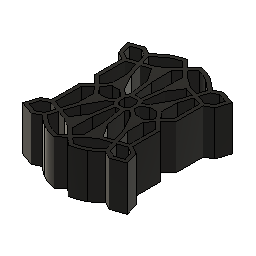
SC-002_shell (Autodesk Fusion 360 design; units mm, degrees)
Autodesk Fusion 360 part; units mm, degrees
sketch "Sketch1" plane through (0, 0, 0) normal (0, 1, 0) x (1, 0, 0)
  line L0 (-3.2742, 2.0082) -> (-1.6589, 0.7858)
  line L1 (-1.6589, 0.7858) -> (-1.6153, -0.6985)
  line L2 (-1.6153, -0.6985) -> (-3.1869, -1.8336)
  line L3 (-3.1869, -1.8336) -> (-5.1951, -1.8336)
  line L4 (-5.1951, -1.8336) -> (-6.8977, 0)
  line L5 (-6.8977, 0) -> (-5.1951, 2.0082)
  line L6 (-5.1951, 2.0082) -> (-3.2742, 2.0082)
  line L7 (3.2742, 2.0082) -> (1.6589, 0.7858)
  line L8 (1.6589, 0.7858) -> (1.6153, -0.6985)
  line L9 (1.6153, -0.6985) -> (3.1869, -1.8336)
  line L10 (3.1869, -1.8336) -> (5.1951, -1.8336)
  line L11 (5.1951, -1.8336) -> (6.8977, 0)
  line L12 (6.8977, 0) -> (5.1951, 2.0082)
  line L13 (5.1951, 2.0082) -> (3.2742, 2.0082)
  line L14 (0, 13.0532) -> (-1.7026, 14.7558)
  spline S0 degree 3 poles (-1.7026, 14.7558) (-2.3211, 14.6321) (-3.7632, 14.197) (-4.6712, 13.5334) knots 0 0 0 0 1 1 1 1
  spline S1 degree 3 poles (-4.6712, 13.5334) (-5.5793, 12.8698) (-6.6576, 11.9181) (-7.0723, 11.5252) knots 0 0 0 0 1 1 1 1
  line L15 (-7.0723, 11.5252) -> (-6.3302, 8.9932)
  line L16 (-6.3302, 8.9932) -> (-3.7544, 9.8663)
  line L17 (-3.7544, 9.8663) -> (-1.7026, 11.3506)
  line L18 (-1.7026, 11.3506) -> (0, 13.0532)
  line L19 (0, 13.0532) -> (1.7026, 14.7558)
  spline S2 degree 3 poles (1.7026, 14.7558) (2.3211, 14.6321) (3.7632, 14.197) (4.6712, 13.5334) knots 0 0 0 0 1 1 1 1
  spline S3 degree 3 poles (4.6712, 13.5334) (5.5793, 12.8698) (6.6576, 11.9181) (7.0723, 11.5252) knots 0 0 0 0 1 1 1 1
  line L20 (7.0723, 11.5252) -> (6.3302, 8.9932)
  line L21 (6.3302, 8.9932) -> (3.7544, 9.8663)
  line L22 (3.7544, 9.8663) -> (1.7026, 11.3506)
  line L23 (1.7026, 11.3506) -> (0, 13.0532)
  line L24 (0, -12.8786) -> (-1.7026, -14.4939)
  spline S4 degree 3 poles (-1.7026, -14.4939) (-2.3211, -14.3702) (-3.689, -14.0355) (-4.6712, -13.4462) knots 0 0 0 0 1 1 1 1
  spline S5 degree 3 poles (-4.6712, -13.4462) (-5.6356, -12.8675) (-6.6576, -11.9182) (-7.0723, -11.5253) knots 0 0 0 0 1 1 1 1
  line L25 (-7.0723, -11.5253) -> (-6.3302, -8.9932)
  line L26 (-6.3302, -8.9932) -> (-3.7544, -9.8663)
  line L27 (-3.7544, -9.8663) -> (-1.7026, -11.176)
  line L28 (-1.7026, -11.176) -> (0, -12.8786)
  line L29 (0, -12.8786) -> (1.7026, -14.4939)
  spline S6 degree 3 poles (1.7026, -14.4939) (2.3211, -14.3702) (3.689, -14.0355) (4.6712, -13.4462) knots 0 0 0 0 1 1 1 1
  spline S7 degree 3 poles (4.6712, -13.4462) (5.6356, -12.8675) (6.6576, -11.9182) (7.0723, -11.5253) knots 0 0 0 0 1 1 1 1
  line L30 (7.0723, -11.5253) -> (6.3302, -8.9932)
  line L31 (6.3302, -8.9932) -> (3.7544, -9.8663)
  line L32 (3.7544, -9.8663) -> (1.7026, -11.176)
  line L33 (1.7026, -11.176) -> (0, -12.8786)
  line L34 (0, 13.0532) -> (-1.7026, 11.3506)
  line L35 (-1.7026, 11.3506) -> (-1.6153, 6.5921)
  line L36 (-1.6153, 6.5921) -> (-1.0041, 1.9645)
  line L37 (-1.0041, 1.9645) -> (0, 1.9645)
  line L38 (0, 1.9645) -> (1.0041, 1.9645)
  line L39 (1.0041, 1.9645) -> (1.6153, 6.5921)
  line L40 (1.6153, 6.5921) -> (1.7026, 11.3506)
  line L41 (1.7026, 11.3506) -> (0, 13.0532)
  line L42 (0, -12.8786) -> (-1.7026, -11.176)
  line L43 (-1.7026, -11.176) -> (-1.6153, -6.5921)
  line L44 (-1.6153, -6.5921) -> (-0.8731, -1.7899)
  line L45 (-0.8731, -1.7899) -> (0, -1.7899)
  line L46 (0, -1.7899) -> (0.8731, -1.7899)
  line L47 (0.8731, -1.7899) -> (1.6153, -6.5921)
  line L48 (1.6153, -6.5921) -> (1.7026, -11.176)
  line L49 (1.7026, -11.176) -> (0, -12.8786)
  line L50 (0, 1.9645) -> (-1.0041, 1.9645)
  line L51 (-1.0041, 1.9645) -> (-1.6589, 0.7858)
  line L52 (-1.6589, 0.7858) -> (-1.6153, -0.6985)
  line L53 (-1.6153, -0.6985) -> (-0.8731, -1.7899)
  line L54 (-0.8731, -1.7899) -> (0, -1.7899)
  line L55 (0, -1.7899) -> (0.8731, -1.7899)
  line L56 (0.8731, -1.7899) -> (1.6153, -0.6985)
  line L57 (1.6153, -0.6985) -> (1.6589, 0.7858)
  line L58 (1.6589, 0.7858) -> (1.0041, 1.9645)
  line L59 (1.0041, 1.9645) -> (0, 1.9645)
  line L60 (-1.6589, 0.7858) -> (-1.0041, 1.9645)
  line L61 (-1.0041, 1.9645) -> (-1.6153, 6.5921)
  line L62 (-1.6153, 6.5921) -> (-3.7544, 9.8663)
  line L63 (-3.7544, 9.8663) -> (-6.3302, 8.9932)
  line L64 (-6.3302, 8.9932) -> (-5.2388, 5.6316)
  line L65 (-5.2388, 5.6316) -> (-3.2742, 2.0082)
  line L66 (-3.2742, 2.0082) -> (-1.6589, 0.7858)
  line L67 (1.6589, 0.7858) -> (1.0041, 1.9645)
  line L68 (1.0041, 1.9645) -> (1.6153, 6.5921)
  line L69 (1.6153, 6.5921) -> (3.7544, 9.8663)
  line L70 (3.7544, 9.8663) -> (6.3302, 8.9932)
  line L71 (6.3302, 8.9932) -> (5.2387, 5.6316)
  line L72 (5.2387, 5.6316) -> (3.2742, 2.0082)
  line L73 (3.2742, 2.0082) -> (1.6589, 0.7858)
  line L74 (-1.6153, -0.6985) -> (-0.8731, -1.7899)
  line L75 (-0.8731, -1.7899) -> (-1.6153, -6.5921)
  line L76 (-1.6153, -6.5921) -> (-3.7544, -9.8663)
  line L77 (-3.7544, -9.8663) -> (-6.3302, -8.9932)
  line L78 (-6.3302, -8.9932) -> (-5.2388, -5.6317)
  line L79 (-5.2388, -5.6317) -> (-3.1869, -1.8336)
  line L80 (-3.1869, -1.8336) -> (-1.6153, -0.6985)
  line L81 (1.6153, -0.6985) -> (0.8731, -1.7899)
  line L82 (0.8731, -1.7899) -> (1.6153, -6.5921)
  line L83 (1.6153, -6.5921) -> (3.7544, -9.8663)
  line L84 (3.7544, -9.8663) -> (6.3302, -8.9932)
  line L85 (6.3302, -8.9932) -> (5.2387, -5.6317)
  line L86 (5.2387, -5.6317) -> (3.1869, -1.8336)
  line L87 (3.1869, -1.8336) -> (1.6153, -0.6985)
  line L88 (-8.8186, 12.442) -> (-7.0723, 11.5252)
  line L89 (-7.0723, 11.5252) -> (-6.3302, 8.9932)
  line L90 (-6.3302, 8.9932) -> (-8.7749, 8.1637)
  line L91 (-8.7749, 8.1637) -> (-10.5212, 9.1241)
  line L92 (-10.5212, 9.1241) -> (-11.307, 11.5689)
  line L93 (-11.307, 11.5689) -> (-8.8186, 12.442)
  line L94 (8.8186, 12.442) -> (7.0723, 11.5252)
  line L95 (7.0723, 11.5252) -> (6.3302, 8.9932)
  line L96 (6.3302, 8.9932) -> (8.7749, 8.1637)
  line L97 (8.7749, 8.1637) -> (10.5212, 9.1241)
  line L98 (10.5212, 9.1241) -> (11.307, 11.5689)
  line L99 (11.307, 11.5689) -> (8.8186, 12.442)
  line L100 (-8.8186, -12.4421) -> (-7.0723, -11.5253)
  line L101 (-7.0723, -11.5253) -> (-6.3302, -8.9932)
  line L102 (-6.3302, -8.9932) -> (-8.7749, -8.1637)
  line L103 (-8.7749, -8.1637) -> (-10.5212, -9.1242)
  line L104 (-10.5212, -9.1242) -> (-11.307, -11.5689)
  line L105 (-11.307, -11.5689) -> (-8.8186, -12.4421)
  line L106 (8.8186, -12.4421) -> (7.0723, -11.5253)
  line L107 (7.0723, -11.5253) -> (6.3302, -8.9932)
  line L108 (6.3302, -8.9932) -> (8.7749, -8.1637)
  line L109 (8.7749, -8.1637) -> (10.5212, -9.1242)
  line L110 (10.5212, -9.1242) -> (11.307, -11.5689)
  line L111 (11.307, -11.5689) -> (8.8186, -12.4421)
  line L112 (-8.7749, 8.1637) -> (-6.3302, 8.9932)
  line L113 (-6.3302, 8.9932) -> (-5.2388, 5.6316)
  line L114 (-5.2388, 5.6316) -> (-5.1951, 2.0082)
  line L115 (-5.1951, 2.0082) -> (-6.8977, 0)
  line L116 (-6.8977, 0) -> (-8.7749, 1.9208)
  line L117 (-8.7749, 1.9208) -> (-8.7749, 8.1637)
  line L118 (8.7749, 8.1637) -> (6.3302, 8.9932)
  line L119 (6.3302, 8.9932) -> (5.2387, 5.6316)
  line L120 (5.2387, 5.6316) -> (5.1951, 2.0082)
  line L121 (5.1951, 2.0082) -> (6.8977, 0)
  line L122 (6.8977, 0) -> (8.7749, 1.9208)
  line L123 (8.7749, 1.9208) -> (8.7749, 8.1637)
  line L124 (-8.7749, -8.1637) -> (-6.3302, -8.9932)
  line L125 (-6.3302, -8.9932) -> (-5.2388, -5.6317)
  line L126 (-5.2388, -5.6317) -> (-5.1951, -1.8336)
  line L127 (-5.1951, -1.8336) -> (-6.8977, 0)
  line L128 (-6.8977, 0) -> (-8.7749, -1.9209)
  line L129 (-8.7749, -1.9209) -> (-8.7749, -8.1637)
  line L130 (8.7749, -8.1637) -> (6.3302, -8.9932)
  line L131 (6.3302, -8.9932) -> (5.2387, -5.6317)
  line L132 (5.2387, -5.6317) -> (5.1951, -1.8336)
  line L133 (5.1951, -1.8336) -> (6.8977, 0)
  line L134 (6.8977, 0) -> (8.7749, -1.9209)
  line L135 (8.7749, -1.9209) -> (8.7749, -8.1637)
  line L136 (0, 0) -> (0, 13.0532)
  constraint coincident L136.start origin
sketch "Sketch2" plane through (0, 0, 0) normal (0, 1, 0) x (1, 0, 0)
  line L0 (0, 0) -> (0, 15)
  line L1 (7.5, 15) -> (-7.5, 15)
  line L2 (-7.5, 15) -> (-7.5, -15)
  line L3 (-7.5, -15) -> (7.5, -15)
  line L4 (7.5, -15) -> (7.5, 15)
  line L5 (7.5, 15) -> (-7.5, -15) construction
  line L6 (-7.5, 15) -> (7.5, -15) construction
  dimension "d2" = 15
  dimension "d4" = 15
  dimension "d5" = 30
  constraint coincident L0.start origin
  constraint vertical L0
  constraint horizontal L1
  constraint perpendicular L1 L2
  constraint parallel L1 L3
  constraint parallel L2 L4
  constraint coincident L5 L0.start
  constraint coincident L6 L0.start
  measures "d2" distance of L0.start L0.end
  measures "d4" distance of L2.end L3.end
  measures "d5" distance of L1.end L2.end
scale "Scale1" [no effect]
sketch "Sketch3" plane through (0, 0, 0) normal (0, 1, 0) x (1, 0, 0)
  line L0 (-11.307, 11.5689) -> (-8.8186, 12.442)
  line L1 (-8.8186, 12.442) -> (-7.0723, 11.5252)
  spline S0 degree 3 poles (-4.6712, 13.5334) (-5.5793, 12.8698) (-6.6576, 11.9181) (-7.0723, 11.5252) knots 0 0 0 0 1 1 1 1
  spline S1 degree 3 poles (-1.7026, 14.7558) (-2.3211, 14.6321) (-3.7632, 14.197) (-4.6712, 13.5334) knots 0 0 0 0 1 1 1 1
  line L2 (0, 13.0532) -> (-1.7026, 14.7558)
  line L3 (0, 13.0532) -> (1.7026, 14.7558)
  spline S2 degree 3 poles (1.7026, 14.7558) (2.3211, 14.6321) (3.7632, 14.197) (4.6712, 13.5334) knots 0 0 0 0 1 1 1 1
  spline S3 degree 3 poles (4.6712, 13.5334) (5.5793, 12.8698) (6.6576, 11.9181) (7.0723, 11.5252) knots 0 0 0 0 1 1 1 1
  line L4 (8.8186, 12.442) -> (7.0723, 11.5252)
  line L5 (11.307, 11.5689) -> (8.8186, 12.442)
  line L6 (10.5212, 9.1241) -> (11.307, 11.5689)
  line L7 (8.7749, 8.1637) -> (10.5212, 9.1241)
  line L8 (8.7749, 1.9208) -> (8.7749, 8.1637)
  line L9 (6.8977, 0) -> (8.7749, 1.9208)
  line L10 (6.8977, 0) -> (8.7749, -1.9209)
  line L11 (8.7749, -1.9209) -> (8.7749, -8.1637)
  line L12 (8.7749, -8.1637) -> (10.5212, -9.1242)
  line L13 (10.5212, -9.1242) -> (11.307, -11.5689)
  line L14 (11.307, -11.5689) -> (8.8186, -12.4421)
  line L15 (8.8186, -12.4421) -> (7.0723, -11.5253)
  spline S4 degree 3 poles (4.6712, -13.4462) (5.6356, -12.8675) (6.6576, -11.9182) (7.0723, -11.5253) knots 0 0 0 0 1 1 1 1
  spline S5 degree 3 poles (1.7026, -14.4939) (2.3211, -14.3702) (3.689, -14.0355) (4.6712, -13.4462) knots 0 0 0 0 1 1 1 1
  line L16 (0, -12.8786) -> (1.7026, -14.4939)
  line L17 (0, -12.8786) -> (-1.7026, -14.4939)
  spline S6 degree 3 poles (-1.7026, -14.4939) (-2.3211, -14.3702) (-3.689, -14.0355) (-4.6712, -13.4462) knots 0 0 0 0 1 1 1 1
  spline S7 degree 3 poles (-4.6712, -13.4462) (-5.6356, -12.8675) (-6.6576, -11.9182) (-7.0723, -11.5253) knots 0 0 0 0 1 1 1 1
  line L18 (-8.8186, -12.4421) -> (-7.0723, -11.5253)
  line L19 (-11.307, -11.5689) -> (-8.8186, -12.4421)
  line L20 (-10.5212, -9.1242) -> (-11.307, -11.5689)
  line L21 (-8.7749, -8.1637) -> (-10.5212, -9.1242)
  line L22 (-8.7749, -1.9209) -> (-8.7749, -8.1637)
  line L23 (-6.8977, 0) -> (-8.7749, -1.9209)
  line L24 (-6.8977, 0) -> (-8.7749, 1.9208)
  line L25 (-8.7749, 1.9208) -> (-8.7749, 8.1637)
  line L26 (-8.7749, 8.1637) -> (-10.5212, 9.1241)
  line L27 (-10.5212, 9.1241) -> (-11.307, 11.5689)
  line L28 (-8.7749, 8.1637) -> (-6.3302, 8.9932)
  line L29 (-7.0723, 11.5252) -> (-6.3302, 8.9932)
  line L30 (-6.3302, 8.9932) -> (-3.7544, 9.8663)
  line L31 (-3.7544, 9.8663) -> (-1.7026, 11.3506)
  line L32 (0, 13.0532) -> (-1.7026, 11.3506)
  line L33 (1.7026, 11.3506) -> (0, 13.0532)
  line L34 (3.7544, 9.8663) -> (1.7026, 11.3506)
  line L35 (3.7544, 9.8663) -> (6.3302, 8.9932)
  line L36 (7.0723, 11.5252) -> (6.3302, 8.9932)
  line L37 (6.3302, 8.9932) -> (8.7749, 8.1637)
  line L38 (6.3302, -8.9932) -> (8.7749, -8.1637)
  line L39 (7.0723, -11.5253) -> (6.3302, -8.9932)
  line L40 (3.7544, -9.8663) -> (6.3302, -8.9932)
  line L41 (3.7544, -9.8663) -> (1.7026, -11.176)
  line L42 (1.7026, -11.176) -> (0, -12.8786)
  line L43 (0, -12.8786) -> (-1.7026, -11.176)
  line L44 (-3.7544, -9.8663) -> (-1.7026, -11.176)
  line L45 (-3.7544, -9.8663) -> (-6.3302, -8.9932)
  line L46 (-7.0723, -11.5253) -> (-6.3302, -8.9932)
  line L47 (-6.3302, -8.9932) -> (-8.7749, -8.1637)
  line L48 (-6.3302, -8.9932) -> (-5.2388, -5.6317)
  line L49 (-5.2388, -5.6317) -> (-3.1869, -1.8336)
  line L50 (-5.2388, -5.6317) -> (-5.1951, -1.8336)
  line L51 (-5.1951, -1.8336) -> (-6.8977, 0)
  line L52 (-3.1869, -1.8336) -> (-5.1951, -1.8336)
  line L53 (-5.1951, 2.0082) -> (-6.8977, 0)
  line L54 (-5.2388, 5.6316) -> (-5.1951, 2.0082)
  line L55 (-6.3302, 8.9932) -> (-5.2388, 5.6316)
  line L56 (-5.1951, 2.0082) -> (-3.2742, 2.0082)
  line L57 (-5.2388, 5.6316) -> (-3.2742, 2.0082)
  line L58 (-3.2742, 2.0082) -> (-1.6589, 0.7858)
  line L59 (-1.0041, 1.9645) -> (-1.6153, 6.5921)
  line L60 (-1.6153, 6.5921) -> (-3.7544, 9.8663)
  line L61 (-1.7026, 11.3506) -> (-1.6153, 6.5921)
  line L62 (1.6153, 6.5921) -> (1.7026, 11.3506)
  line L63 (1.6153, 6.5921) -> (3.7544, 9.8663)
  line L64 (6.3302, 8.9932) -> (5.2387, 5.6316)
  line L65 (5.2387, 5.6316) -> (5.1951, 2.0082)
  line L66 (5.1951, 2.0082) -> (6.8977, 0)
  line L67 (5.1951, -1.8336) -> (6.8977, 0)
  line L68 (5.2387, -5.6317) -> (5.1951, -1.8336)
  line L69 (6.3302, -8.9932) -> (5.2387, -5.6317)
  line L70 (1.6153, -6.5921) -> (3.7544, -9.8663)
  line L71 (1.6153, -6.5921) -> (1.7026, -11.176)
  line L72 (-1.7026, -11.176) -> (-1.6153, -6.5921)
  line L73 (-1.6153, -6.5921) -> (-3.7544, -9.8663)
  line L74 (-1.6153, -6.5921) -> (-0.8731, -1.7899)
  line L75 (0.8731, -1.7899) -> (1.6153, -6.5921)
  line L76 (5.2387, -5.6317) -> (3.1869, -1.8336)
  line L77 (3.1869, -1.8336) -> (5.1951, -1.8336)
  line L78 (0, -1.7899) -> (0.8731, -1.7899)
  line L79 (-1.6153, -0.6985) -> (-3.1869, -1.8336)
  line L80 (-1.6153, -0.6985) -> (-0.8731, -1.7899)
  line L81 (-0.8731, -1.7899) -> (0, -1.7899)
  line L82 (0.8731, -1.7899) -> (1.6153, -0.6985)
  line L83 (1.6153, -0.6985) -> (3.1869, -1.8336)
  line L84 (1.6589, 0.7858) -> (1.6153, -0.6985)
  line L85 (-1.6589, 0.7858) -> (-1.6153, -0.6985)
  line L86 (-1.6589, 0.7858) -> (-1.0041, 1.9645)
  line L87 (0, 1.9645) -> (-1.0041, 1.9645)
  line L88 (1.0041, 1.9645) -> (0, 1.9645)
  line L89 (1.6589, 0.7858) -> (1.0041, 1.9645)
  line L90 (1.0041, 1.9645) -> (1.6153, 6.5921)
  line L91 (3.2742, 2.0082) -> (1.6589, 0.7858)
  line L92 (5.1951, 2.0082) -> (3.2742, 2.0082)
  line L93 (5.2387, 5.6316) -> (3.2742, 2.0082)
  line L94 (-7.4085, 11.2499) -> (-6.8219, 9.2487)
  line L95 (-8.7365, 8.5991) -> (-6.8219, 9.2487)
  line L96 (-8.7365, 8.5991) -> (-10.189, 9.398)
  line L97 (-10.189, 9.398) -> (-10.807, 11.3204)
  line L98 (-10.807, 11.3204) -> (-8.8504, 12.0069)
  line L99 (-8.8504, 12.0069) -> (-7.4085, 11.2499)
  line L100 (-0.5657, 13.0532) -> (-1.9629, 11.656)
  line L101 (-3.94, 10.2257) -> (-1.9629, 11.656)
  line L102 (-6.0636, 9.5059) -> (-3.94, 10.2257)
  line L103 (-6.6189, 11.4005) -> (-6.0636, 9.5059)
  spline S8 degree 3 poles (-4.4352, 13.2105) (-5.2085, 12.6454) (-6.1342, 11.8442) (-6.6189, 11.4005) knots 0 0 0 0 0.875986 0.875986 0.875986 0.875986
  spline S9 degree 3 poles (-1.8301, 14.3176) (-2.4821, 14.1594) (-3.7085, 13.7415) (-4.4352, 13.2105) knots 0.105546 0.105546 0.105546 0.105546 1 1 1 1
  line L104 (-0.5657, 13.0532) -> (-1.8301, 14.3176)
  line L105 (1.9629, 11.656) -> (0.5657, 13.0532)
  line L106 (0.5657, 13.0532) -> (1.8301, 14.3176)
  spline S10 degree 3 poles (1.8301, 14.3176) (2.4821, 14.1594) (3.7085, 13.7415) (4.4352, 13.2105) knots 0.105546 0.105546 0.105546 0.105546 1 1 1 1
  spline S11 degree 3 poles (4.4352, 13.2105) (5.2085, 12.6454) (6.1342, 11.8442) (6.6189, 11.4005) knots 0 0 0 0 0.875986 0.875986 0.875986 0.875986
  line L107 (6.6189, 11.4005) -> (6.0636, 9.5059)
  line L108 (3.94, 10.2257) -> (6.0636, 9.5059)
  line L109 (3.94, 10.2257) -> (1.9629, 11.656)
  line L110 (6.8219, 9.2487) -> (8.7365, 8.5991)
  line L111 (8.7365, 8.5991) -> (10.189, 9.398)
  line L112 (10.189, 9.398) -> (10.8069, 11.3204)
  line L113 (10.8069, 11.3204) -> (8.8504, 12.0069)
  line L114 (8.8504, 12.0069) -> (7.4084, 11.2499)
  line L115 (7.4084, 11.2499) -> (6.8219, 9.2487)
  line L116 (6.5854, 8.4841) -> (8.3749, 7.877)
  line L117 (8.3749, 2.0838) -> (8.3749, 7.877)
  line L118 (6.9187, 0.5938) -> (8.3749, 2.0838)
  line L119 (5.5969, 2.1528) -> (6.9187, 0.5938)
  line L120 (5.638, 5.566) -> (5.5969, 2.1528)
  line L121 (6.5854, 8.4841) -> (5.638, 5.566)
  line L122 (1.418, 2.0432) -> (1.9999, 6.4495)
  line L123 (1.9999, 6.4495) -> (3.9197, 9.3879)
  line L124 (3.9197, 9.3879) -> (5.8278, 8.7411)
  line L125 (5.8278, 8.7411) -> (4.8696, 5.79)
  line L126 (4.8696, 5.79) -> (2.9638, 2.2749)
  line L127 (2.9638, 2.2749) -> (1.7849, 1.3827)
  line L128 (1.7849, 1.3827) -> (1.418, 2.0432)
  line L129 (1.2995, 11.188) -> (0, 12.4875)
  line L130 (0, 12.4875) -> (-1.2995, 11.188)
  line L131 (-1.2995, 11.188) -> (-1.2158, 6.622)
  line L132 (-0.6535, 2.3645) -> (-1.2158, 6.622)
  line L133 (0, 2.3645) -> (-0.6535, 2.3645)
  line L134 (0.6534, 2.3645) -> (0, 2.3645)
  line L135 (0.6534, 2.3645) -> (1.2158, 6.622)
  line L136 (1.2158, 6.622) -> (1.2995, 11.188)
  line L137 (-1.2559, 0.6876) -> (-0.7687, 1.5645)
  line L138 (0, 1.5645) -> (-0.7687, 1.5645)
  line L139 (0.7687, 1.5645) -> (0, 1.5645)
  line L140 (1.2559, 0.6876) -> (0.7687, 1.5645)
  line L141 (1.2559, 0.6876) -> (1.2189, -0.5701)
  line L142 (0.6614, -1.3899) -> (1.2189, -0.5701)
  line L143 (0, -1.3899) -> (0.6614, -1.3899)
  line L144 (-0.6614, -1.3899) -> (0, -1.3899)
  line L145 (-1.2189, -0.5701) -> (-0.6614, -1.3899)
  line L146 (-1.2559, 0.6876) -> (-1.2189, -0.5701)
  line L147 (-1.9999, 6.4495) -> (-3.9197, 9.3879)
  line L148 (-5.8278, 8.7411) -> (-3.9197, 9.3879)
  line L149 (-5.8278, 8.7411) -> (-4.8696, 5.79)
  line L150 (-4.8696, 5.79) -> (-2.9638, 2.2749)
  line L151 (-2.9638, 2.2749) -> (-1.7849, 1.3827)
  line L152 (-1.7849, 1.3827) -> (-1.418, 2.0432)
  line L153 (-1.418, 2.0432) -> (-1.9999, 6.4495)
  line L154 (-6.5854, 8.4841) -> (-5.638, 5.566)
  line L155 (-5.638, 5.566) -> (-5.5969, 2.1528)
  line L156 (-5.5969, 2.1528) -> (-6.9187, 0.5938)
  line L157 (-6.9187, 0.5938) -> (-8.3749, 2.0838)
  line L158 (-8.3749, 2.0838) -> (-8.3749, 7.877)
  line L159 (-8.3749, 7.877) -> (-6.5854, 8.4841)
  line L160 (-2.0531, 0.5825) -> (-2.0213, -0.4984)
  line L161 (-2.0213, -0.4984) -> (-3.3163, -1.4336)
  line L162 (-3.3163, -1.4336) -> (-5.0207, -1.4336)
  line L163 (-5.0207, -1.4336) -> (-6.363, 0.012)
  line L164 (-5.0098, 1.6082) -> (-6.363, 0.012)
  line L165 (-5.0098, 1.6082) -> (-3.4085, 1.6082)
  line L166 (-3.4085, 1.6082) -> (-2.0531, 0.5825)
  line L167 (5.0098, 1.6082) -> (3.4085, 1.6082)
  line L168 (3.4085, 1.6082) -> (2.0531, 0.5825)
  line L169 (2.0531, 0.5825) -> (2.0213, -0.4984)
  line L170 (2.0213, -0.4984) -> (3.3162, -1.4336)
  line L171 (3.3162, -1.4336) -> (5.0207, -1.4336)
  line L172 (5.0207, -1.4336) -> (6.363, 0.012)
  line L173 (5.0098, 1.6082) -> (6.363, 0.012)
  line L174 (6.9051, -0.5799) -> (8.3749, -2.0839)
  line L175 (8.3749, -2.0839) -> (8.3749, -7.8771)
  line L176 (6.5854, -8.4842) -> (8.3749, -7.8771)
  line L177 (6.5854, -8.4842) -> (5.638, -5.5661)
  line L178 (5.638, -5.5661) -> (5.5969, -1.9887)
  line L179 (5.5969, -1.9887) -> (6.9051, -0.5799)
  line L180 (8.7365, -8.5992) -> (10.189, -9.398)
  line L181 (10.189, -9.398) -> (10.8069, -11.3205)
  line L182 (10.8069, -11.3205) -> (8.8504, -12.007)
  line L183 (8.8504, -12.007) -> (7.4084, -11.25)
  line L184 (7.4084, -11.25) -> (6.8219, -9.2488)
  line L185 (6.8219, -9.2488) -> (8.7365, -8.5992)
  line L186 (3.9288, -10.2296) -> (6.0636, -9.5059)
  line L187 (6.6193, -11.402) -> (6.0636, -9.5059)
  spline S12 degree 3 poles (4.4654, -13.1032) (5.2592, -12.6269) (6.1389, -11.8492) (6.6193, -11.402) knots 0 0 0 0 0.876354 0.876354 0.876354 0.876354
  spline S13 degree 3 poles (1.8257, -14.0593) (2.4857, -13.9142) (3.6571, -13.5882) (4.4654, -13.1032) knots 0.100921 0.100921 0.100921 0.100921 1 1 1 1
  line L188 (0.5732, -12.8711) -> (1.8257, -14.0593)
  line L189 (1.9546, -11.4897) -> (0.5732, -12.8711)
  line L190 (3.9288, -10.2296) -> (1.9546, -11.4897)
  line L191 (-3.9288, -10.2296) -> (-1.9546, -11.4897)
  line L192 (-0.5732, -12.8711) -> (-1.9546, -11.4897)
  line L193 (-0.5732, -12.8711) -> (-1.8257, -14.0593)
  spline S14 degree 3 poles (-1.8257, -14.0593) (-2.4857, -13.9142) (-3.6571, -13.5882) (-4.4654, -13.1032) knots 0.100921 0.100921 0.100921 0.100921 1 1 1 1
  spline S15 degree 3 poles (-4.4654, -13.1032) (-5.2592, -12.6269) (-6.1389, -11.8492) (-6.6194, -11.402) knots 0 0 0 0 0.876354 0.876354 0.876354 0.876354
  line L194 (-6.6194, -11.402) -> (-6.0636, -9.5059)
  line L195 (-3.9288, -10.2296) -> (-6.0636, -9.5059)
  line L196 (-8.7365, -8.5992) -> (-10.189, -9.398)
  line L197 (-10.189, -9.398) -> (-10.807, -11.3205)
  line L198 (-10.807, -11.3205) -> (-8.8504, -12.007)
  line L199 (-8.8504, -12.007) -> (-7.4085, -11.25)
  line L200 (-7.4085, -11.25) -> (-6.8219, -9.2488)
  line L201 (-6.8219, -9.2488) -> (-8.7365, -8.5992)
  line L202 (-6.5854, -8.4842) -> (-8.3749, -7.8771)
  line L203 (-8.3749, -2.0839) -> (-8.3749, -7.8771)
  line L204 (-6.9051, -0.5799) -> (-8.3749, -2.0839)
  line L205 (-5.5969, -1.9887) -> (-6.9051, -0.5799)
  line L206 (-5.638, -5.5661) -> (-5.5969, -1.9887)
  line L207 (-6.5854, -8.4842) -> (-5.638, -5.5661)
  line L208 (-1.7147, -1.2637) -> (-2.8785, -2.1043)
  line L209 (-4.8695, -5.7898) -> (-2.8785, -2.1043)
  line L210 (-5.8278, -8.7412) -> (-4.8695, -5.7898)
  line L211 (-3.9197, -9.388) -> (-5.8278, -8.7412)
  line L212 (-1.9974, -6.4457) -> (-3.9197, -9.388)
  line L213 (-1.9974, -6.4457) -> (-1.2925, -1.8846)
  line L214 (-1.7147, -1.2637) -> (-1.2925, -1.8846)
  line L215 (1.7147, -1.2637) -> (2.8785, -2.1043)
  line L216 (4.8695, -5.7898) -> (2.8785, -2.1043)
  line L217 (5.8278, -8.7412) -> (4.8695, -5.7898)
  line L218 (3.9197, -9.388) -> (5.8278, -8.7412)
  line L219 (1.9974, -6.4457) -> (3.9197, -9.388)
  line L220 (1.2925, -1.8846) -> (1.9974, -6.4457)
  line L221 (1.2925, -1.8846) -> (1.7147, -1.2637)
  line L222 (1.2159, -6.6266) -> (1.2994, -11.0135)
  line L223 (1.2994, -11.0135) -> (0, -12.3129)
  line L224 (0, -12.3129) -> (-1.2994, -11.0135)
  line L225 (-1.2994, -11.0135) -> (-1.2159, -6.6266)
  line L226 (-1.2159, -6.6266) -> (-0.5302, -2.1899)
  line L227 (-0.5302, -2.1899) -> (0, -2.1899)
  line L228 (0, -2.1899) -> (0.5302, -2.1899)
  line L229 (0.5302, -2.1899) -> (1.2159, -6.6266)
  dimension "d6" = 0.4
  dimension "d10" = 0.4
  dimension "d14" = 0.4
  dimension "d15" = 0.4
  dimension "d19" = 0.4
  dimension "d20" = 0.4
  dimension "d22" = 0.4
  dimension "d23" = 0.4
  dimension "d24" = 0.4
  dimension "d25" = 0.4
  dimension "d29" = 0.4
  dimension "d30" = 0.4
extrude "Extrude1" add sketch "Sketch3" along normal blind 10 makes body 1
extrude "Extrude2" add sketch "Sketch3" along normal blind 0.2 separate body contours L94 L95 L96 L97 L98 L99 | L100 L101 L102 L103 S8 S9 L104 | L105 L106 S10 S11 L107 L108 L109 | L110 L111 L112 L113 L114 L115 | L116 L117 L118 L119 L120 L121 | L122 L123 L124 L125 L126 L127 L128 | L129 L130 L131 L132 L133 L134 L135 L136 | L137 L138 L139 L140 L141 L142 L143 L144 L145 L146 | L147 L148 L149 L150 L151 L152 L153 | L154 L155 L156 L157 L158 L159 | L160 L161 L162 L163 L164 L165 L166 | L167 L168 L169 L170 L171 L172 L173 | L174 L175 L176 L177 L178 L179 | L180 L181 L182 L183 L184 L185 | L186 L187 S12 S13 L188 L189 L190 | L191 L192 L193 S14 S15 L194 L195 | L196 L197 L198 L199 L200 L201 | L202 L203 L204 L205 L206 L207 | L208 L209 L210 L211 L212 L213 L214 | L215 L216 L217 L218 L219 L220 L221 | L222 L223 L224 L225 L226 L227 L228 L229 makes body 2 at (-3.2485, 0, 4.7799) makes body 3 at (7.4626, 0, -5.1756) makes body 4 at (0.4053, 0, 9.5512) makes body 5 at (8.778, 0, -9.749) makes body 6 at (-7.4626, 0, -5.1756) makes body 7 at (-7.4626, 0, 5.1757) makes body 8 at (4.998, 0, -11.6122) makes body 9 at (-3.4496, 0, 11.6075) makes body 10 at (3.9151, 0, 0.4197) makes body 11 at (-0.4063, 0, -0.2684) makes body 12 at (-3.9151, 0, 0.4197) makes body 13 at (3.2778, 0, -4.8381) makes body 14 at (3.2485, 0, 4.7799) makes body 15 at (8.778, 0, 9.749) makes body 16 at (-8.778, 0, -9.749) makes body 17 at (-8.778, 0, 9.749) makes body 18 at (-4.998, 0, -11.6122) makes body 19 at (3.4496, 0, 11.6075) makes body 20 at (7.4626, 0, 5.1757) makes body 21 at (-0.4053, 0, -9.666) makes body 22 at (-3.2778, 0, -4.8381)
copy_body "Body->Comp1" bodies 2 removing the originals makes body 23 in component "diffusor"
copy_body "CutPasteBodies1" bodies 3 4 5 6 7 8 9 10 11 12 13 20 14 21 15 22 16 17 18 19 removing the originals makes body 24 makes body 25 makes body 26 makes body 27 makes body 28 makes body 29 makes body 30 makes body 31 makes body 32 makes body 33 makes body 34 makes body 35 makes body 36 makes body 37 makes body 38 makes body 39 makes body 40 makes body 41 makes body 42 makes body 43 in component "diffusor"
move_face "OffsetFaces1" offset 0.4 36 faces at (9.357, 3.3333, -8.4838) (8.7749, 3.3333, -4.0018) (7.5234, 3.3333, -0.6403) (7.5234, 3.3333, 0.6403) (8.7749, 3.3333, 4.0019) (9.357, 3.3333, 8.4839) (10.7831, 3.3333, 9.9391) (10.4775, 3.3333, 11.86) (8.2365, 3.3333, 12.1365) (4.9939, 4.4444, 13.2408) (4.3311, 4.4444, 13.6332) (0.5675, 3.3333, 13.417) (-0.5675, 3.3333, 13.417) (-4.3311, 4.4444, 13.6332) (-4.9939, 4.4444, 13.2408) (-8.2365, 3.3333, 12.1365) (-10.4775, 6.6667, 11.86) (-10.7831, 3.3333, 9.9391) (-9.357, 3.3333, 8.4839) (-8.7749, 3.3333, 4.0019) (-7.5234, 3.3333, 0.6403) (-7.5234, 3.3333, -0.6403) (-8.7749, 3.3333, -4.0018) (-9.357, 3.3333, -8.4838) (-10.7831, 3.3333, -9.939) (-10.4775, 6.6667, -11.8599) (-8.2365, 3.3333, -12.1364) (-6.1993, 8.8889, -12.3059) (-4.3506, 5.5556, -13.746) (-0.5675, 3.3333, -13.6207) (0.5675, 6.6667, -13.6207) (4.3506, 5.5556, -13.746) (6.1993, 8.8889, -12.3059) (8.2365, 3.3333, -12.1364) (10.4775, 6.6667, -11.8599) (10.7831, 3.3333, -9.939) on bodies 1
sketch "Sketch4" plane through (0, 0, 0) normal (0, 1, 0) x (1, 0, 0)
  line L0 (1, 1) -> (-1, 1)
  line L1 (-1, 1) -> (-1, -1)
  line L2 (-1, -1) -> (1, -1)
  line L3 (1, -1) -> (1, 1)
  line L4 (1, 1) -> (-1, -1) construction
  line L5 (-1, 1) -> (1, -1) construction
  dimension "d35" = 2
  dimension "d36" = 2
  constraint horizontal L0
  constraint perpendicular L0 L1
  constraint parallel L0 L2
  constraint parallel L1 L3
  constraint coincident L4 origin
  constraint coincident L5 origin
  measures "d35" distance of L1.end L2.end
  measures "d36" distance of L0.end L1.end
extrude "Extrude3" [suppressed]
copy_body "Body->Comp2" [suppressed] in component "led"
component "diffusor" placed x (1, 0, 0) y (0, 1, 0) z (0, 0, 1) at (0, 9.6, 0)
equation "d6 = segment_pffset"
equation "d9 = -segment_pffset"
equation "d10 = segment_pffset"
equation "wall_size = 0.8 mm"
equation "segment_pffset = wall_size / 2"
equation "d13 = -segment_pffset"
equation "d14 = segment_pffset"
equation "d15 = segment_pffset"
equation "d16 = -segment_pffset"
equation "d17 = -segment_pffset"
equation "d18 = -segment_pffset"
equation "d19 = segment_pffset"
equation "d20 = segment_pffset"
equation "d21 = -segment_pffset"
equation "d22 = segment_pffset"
equation "d23 = segment_pffset"
equation "d24 = segment_pffset"
equation "d25 = segment_pffset"
equation "d26 = -segment_pffset"
equation "d27 = -segment_pffset"
equation "d28 = -segment_pffset"
equation "d29 = segment_pffset"
equation "d30 = segment_pffset"
